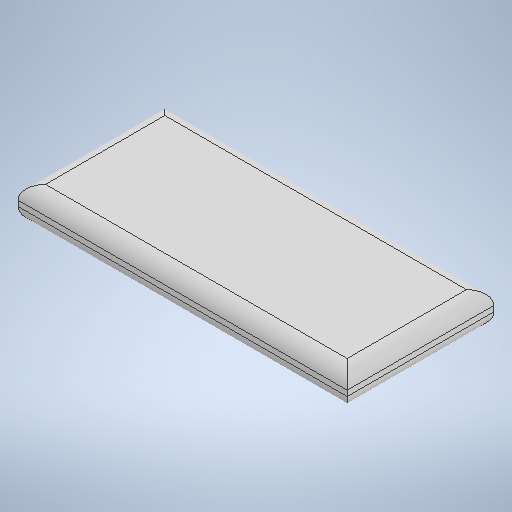
# Autodesk Inventor part: 3,.7V 500mAh
Saved by Autodesk Inventor 2026 (Build 300175050, 175E)
## iProperties
Created: 2025-07-11
Part Number: 3,.7V 500mAh
Material: Generic
Document SubType Name: Modeling
Designer: Jochen Alt
Density: 1 g/cm^3
Appearance: Default
Author: Jochen Alt
Autodesk Inventor part; units mm, degrees
ref_plane "YZ Plane" through (0, 0, 0) normal (1, 0, 0) x (0, 1, 0)
ref_plane "XZ Plane" through (0, 0, 0) normal (0, 1, 0) x (-1, 0, 0)
ref_plane "XY Plane" through (0, 0, 0) normal (0, 0, 1) x (1, 0, 0)
sketch "Sketch1" plane through (0, 0, 0) normal (0, 0, 1) x (1, 0, 0)
  line L0 (0, 14.98) -> (0, -14.98) construction
  line L1 (-33.6, 0) -> (33.6, 0) construction
  line L2 (24, -10.7) -> (-24, -10.7)
  line L3 (-24, -10.7) -> (-24, 10.7)
  line L4 (-24, 10.7) -> (24, 10.7)
  line L5 (24, 10.7) -> (24, -10.7)
  line L6 (24, -10.7) -> (-24, 10.7) construction
  line L7 (-24, -10.7) -> (24, 10.7) construction
  point P0 (0, 0)
  dimension "d0" = 21.4
  dimension "d1" = 48
  constraints: 12 end point, 2 midpoint, 2 parallel, 1 horizontal, 1 perpendicular
  measures "d0" distance of L4.end L2.start
  measures "d1" distance of L3.end L4.end
extrude "Extrusion1" add sketch "Sketch1" along normal blind 4.8
fillet "Fillet1" radius 2 8 edges at (0, -10.7, 4.8) (0, -10.7, 0) (0, 10.7, 4.8) (0, 10.7, 0) (24, 0, 4.8) (24, 0, 0) (-24, 0, 0) (-24, 0, 4.8)
body "Solid1"
